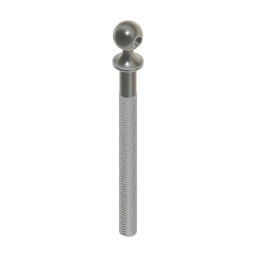
Screw (Autodesk Fusion 360 design; units mm, degrees)
Autodesk Fusion 360 part; units mm, degrees
cylinder "CylinderPrimitive1" add diameter 12.6746 height 150.7998 placed x (1, 0, 0) y (0, 1, 0) z (0, 0, 1) at (0, 0, 0) makes body 1
thread "Thread1" "ANSI Unified Screw Threads 0.5 1/2-12 UNS 3A" major diameter 12.5552 minor diameter 10.1803 pitch 2.1167 angle 60 modelled right hand crest width 0.3192 on face at (6.3058, -0.631, 100.5332) from (0, 0, 0) to (0, 0, 123.825) crest through (6.2776, 0, -0.5292) on bodies 1
sketch "Sketch2" plane through (0, 0, 150.7998) normal (0, 0, 1) x (-1, 0, 0)
  circle A0 centre (0, 0) radius 6.2776
  circle A1 centre (0, 0) radius 11.1125
  circle A2 centre (0, 0) radius 3.81
  dimension "d5" = 22.225
  dimension "d6" = 7.62
  constraint coincident A0.centre A1.centre
  measures "d5" diameter of A1
  measures "d6" diameter of A2
extrude "Extrude1" add sketch "Sketch2" along normal blind 2.2098 separate body contours A1 makes body 2
sketch "Sketch3" plane through (0, 0, 0) normal (0, 1, 0) x (1, 0, 0)
  line L0 (-11.1125, -153.0096) -> (11.1125, -153.0096)
  line L1 (0, -150.7869) -> (0, -165.0617)
  line L2 (0, -165.0617) -> (-3.81, -165.0617)
  arc A0 (-3.81, -165.0617) -> (-11.1125, -153.0096) centre (-16.0531, -164.2416) ccw
  dimension "d9" = 14.2748
  dimension "d10" = 3.81
  constraint perpendicular L0 L1
  constraint perpendicular L1 L2
  measures "d9" distance of L1.start L1.end
  measures "d10" distance of L1.end L2.end
extrude "Extrude2" add 1 faces at (-2.2367, 1.4233, 150.7998) along direction (0, 0, 1) blind 2.2098 on bodies 1 bodies 1 2
revolve "Revolve1" add sketch "Sketch3" angle 360 about axis through (0, 0, 150.7869) along (0, 0, 1) bodies 1
sphere "SpherePrimitive1" add diameter 22.225 placed x (-1, 0, 0) y (0, -1, 0) z (0, 0, 1) at (0, 0, 165.0617) separate body makes body 3
move_body "Move1" bodies 3 to x (1, 0, 0) y (0, 1, 0) z (0, 0, 1) at (0, 0, 16.1357)
sketch "Sketch5" plane through (0, 0, 0) normal (0, 1, 0) x (1, 0, 0)
move_body "Move2" bodies 3 to x (1, 0, 0) y (0, 1, 0) z (0, 0, 1) at (0, 0, -5.6821)
combine "Combine1" operation add target body 3 tool bodies 1
sketch "Sketch6" plane through (0, 0, 0) normal (1, 0, 0) x (0, 1, 0)
  circle A0 centre (0, 175.26) radius 4.3561
  dimension "d15" = 8.7122
  measures "d15" diameter of A0
extrude "Extrude3" cut sketch "Sketch6" along normal mid plane 50.8 bodies 3
